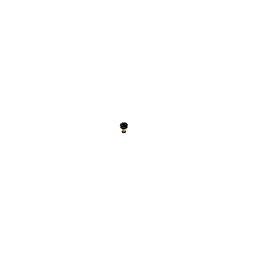
shadowmask_LN_evap_fixture (Autodesk Fusion 360 archive; units mm, degrees)
design "pelco_SEMclip_simplified_bolt"
Autodesk Fusion 360 part; units mm, degrees
sketch "Sketch3" plane through (0, 0, 1.43) normal (0, 0, 1) x (-1, 0, 0)
  circle A0 centre (0, 0) radius 1.895
  line L0 (-2, -0.3) -> (2, -0.3)
  line L1 (2, -0.3) -> (2, 0.3)
  line L2 (2, 0.3) -> (-2, 0.3)
  line L3 (-2, 0.3) -> (-2, -0.3)
  line L4 (-2, -0.3) -> (2, 0.3) construction
  line L5 (2, -0.3) -> (-2, 0.3) construction
  constraint horizontal L0
  constraint perpendicular L0 L1
  constraint parallel L0 L2
  constraint parallel L1 L3
  constraint coincident L4 A0.centre
  constraint coincident L5 A0.centre
  constraint coincident A0.centre origin
sketch "Sketch1" plane through (0, 0, 0.2) normal (0, 0, 1) x (-1, 0, 0)
  line L0 (1.6, -1.9) -> (1.6, -0.0323)
  line L1 (1.6, -0.0323) -> (1.5997, -0.0323)
  arc A0 (1.5997, -0.0323) -> (-1.5997, -0.0323) centre (0, 0) ccw
  line L2 (-1.5997, -0.0323) -> (-1.6, -0.0323)
  line L3 (-1.6, -0.0323) -> (-1.6, -1.9)
  line L4 (-1.6, -1.9) -> (1.6, -1.9)
  circle A1 centre (0, 0) radius 1.05
  circle A2 centre (0, 0) radius 1.895
  dimension "d39" = 3.79
  constraint concentric A0 A2
  measures "d39" diameter of A2
extrude "Extrude1" add sketch "Sketch1" along normal blind 1.23 contours L0 A0 L3 A2 | L0 A0 L3 A2 | A1
sketch "Sketch2" plane through (0, 0, 0.2) normal (0, 0, -1) x (1, 0, 0)
  circle A0 centre (0, 0) radius 1.895
  circle A1 centre (0, 0) radius 1
  dimension "d42" = 2
  constraint coincident A0.centre A1.centre
  measures "d42" diameter of A1
extrude "Extrude2" add sketch "Sketch2" along normal blind 3.5 contours A1
extrude "Extrude3" cut sketch "Sketch3" against normal blind 1 contours A0 L0 L2

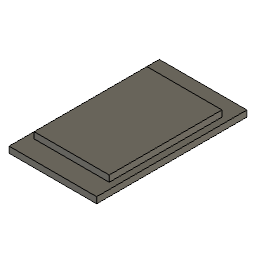
design "6x9_12x7_300um_sm_flipchip_assemb"
Autodesk Fusion 360 part; units mm, degrees
sketch "Sketch1" plane through (0, 0, 0) normal (0, 0, 1) x (1, 0, 0)
  line L0 (3.5, 6) -> (-3.5, 6)
  line L1 (-3.5, 6) -> (-3.5, -6)
  line L2 (-3.5, -6) -> (3.5, -6)
  line L3 (3.5, -6) -> (3.5, 6)
  line L4 (3.5, 6) -> (-3.5, -6) construction
  line L5 (-3.5, 6) -> (3.5, -6) construction
  dimension "d1" = 7
  dimension "d2" = 12
  constraint horizontal L0
  constraint perpendicular L0 L1
  constraint parallel L0 L2
  constraint parallel L1 L3
  constraint coincident L4 origin
  constraint coincident L5 origin
  measures "d1" distance of L1 L3
  measures "d2" distance of L0 L2
extrude "Extrude1" add sketch "Sketch1" along normal blind 0.5 makes body 1
sketch "Sketch2" plane through (0, 0, 0) normal (0, 0, -1) x (1, 0, 0)
  line L0 (3.5, -6) -> (3.5, 6)
  line L1 (3.5, 6) -> (-3.5, 6)
  line L2 (-3.5, 6) -> (-3.5, -6)
  line L3 (-3.5, -6) -> (3.5, -6)
  line L4 (2, 2.5) -> (-2, 2.5)
  line L5 (-2, 2.5) -> (-2, -2.5)
  line L6 (-2, -2.5) -> (2, -2.5)
  line L7 (2, -2.5) -> (2, 2.5)
  line L8 (2, 2.5) -> (-2, -2.5) construction
  line L9 (-2, 2.5) -> (2, -2.5) construction
  dimension "d6" = 4
  dimension "d7" = 5
  constraint horizontal L4
  constraint perpendicular L4 L5
  constraint parallel L4 L6
  constraint parallel L5 L7
  constraint coincident L8 origin
  constraint coincident L9 origin
  measures "d6" distance of L5 L7
  measures "d7" distance of L4 L6
extrude "Extrude2" cut sketch "Sketch2" against normal blind 0.25 contours L4 L5 L6 L7 bodies 1
chamfer "Chamfer2" distance 0.25 angle 45 4 edges at (-2, 0, 0.25) (0, 2.5, 0.25) (0, -2.5, 0.25) (2, 0, 0.25) on bodies 1
sketch "Sketch3" plane through (0, 0, 0.5) normal (0, 0, 1) x (-1, 0, 0)
  line L0 (-3.5, -6) -> (3.5, -6)
  line L1 (3.5, -6) -> (3.5, 6)
  line L2 (3.5, 6) -> (-3.5, 6)
  line L3 (-3.5, 6) -> (-3.5, -6)
  line L4 (-3, -4.5) -> (3, -4.5)
  line L5 (3, -4.5) -> (3, 4.5)
  line L6 (3, 4.5) -> (-3, 4.5)
  line L7 (-3, 4.5) -> (-3, -4.5)
  line L8 (-3, -4.5) -> (3, 4.5) construction
  line L9 (3, -4.5) -> (-3, 4.5) construction
  dimension "d11" = 9
  dimension "d12" = 6
  constraint horizontal L4
  constraint perpendicular L4 L5
  constraint parallel L4 L6
  constraint parallel L5 L7
  constraint coincident L8 origin
  constraint coincident L9 origin
  measures "d11" distance of L4.end L5.end
  measures "d12" distance of L4.start L4.end
extrude "Extrude3" add sketch "Sketch3" along normal blind 0.5 contours L4 L5 L6 L7 bodies 1
sketch "Sketch4" plane through (0, 0, 0.25) normal (0, 0, -1) x (1, 0, 0)
  line L0 (-1.75, -2.25) -> (1.75, -2.25)
  line L1 (1.75, -2.25) -> (1.75, 2.25)
  line L2 (1.75, 2.25) -> (-1.75, 2.25)
  line L3 (-1.75, 2.25) -> (-1.75, -2.25)
  line L4 (1.75, -2.25) -> (-1.75, -2.25)
  line L5 (-1.75, -2.25) -> (-1.75, 2.25)
  line L6 (-1.75, 2.25) -> (1.75, 2.25)
  line L7 (1.75, 2.25) -> (1.75, -2.25)
  constraint horizontal L4
  constraint vertical L5
  constraint horizontal L6
  constraint vertical L7
  constraint coincident L2.end L3.start
  constraint coincident L0.end L1.start
extrude "Extrude4" add sketch "Sketch4" along normal blind 0.01 from surface at 0.01 separate body makes body 2

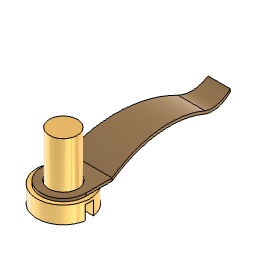
design "pelco_SEMclip_simplified_flipped"
Autodesk Fusion 360 part; units mm, degrees
sketch "Sketch1" plane through (0, 0, 0) normal (0, 0, 1) x (1, 0, 0)
  circle A0 centre (0, 0) radius 1.05
  circle A1 centre (0, 0) radius 1.6
  line L0 (-1.6, 1.9) -> (1.6, 1.9)
  line L1 (1.6, 1.9) -> (1.6, 0.0323)
  line L2 (1.6, 0.0323) -> (-1.6, 0.0323)
  line L3 (-1.6, 0.0323) -> (-1.6, 1.9)
  line L4 (-0.8, 11.2) -> (0.8, 11.2)
  line L5 (0.8, 11.2) -> (0.8, 10.2)
  line L6 (0.8, 10.2) -> (-0.8, 10.2)
  line L7 (-0.8, 10.2) -> (-0.8, 11.2)
  line L8 (-1.6, 1.9) -> (-0.8, 11.2)
  line L9 (0.8, 11.2) -> (1.6, 1.9)
  dimension "d1" = 2.1
  dimension "d2" = 3.2
  dimension "d3" = 1.6
  dimension "d4" = 1.6
  dimension "d5" = 1.9
  dimension "d6" = 0.8
  dimension "d7" = 0.8
  dimension "d8" = 11.2
  constraint coincident A0.centre A1.centre
  constraint concentric A0 A1
  constraint horizontal L0
  constraint vertical L1
  constraint horizontal L2
  constraint vertical L3
  constraint horizontal L4
  constraint vertical L5
  constraint horizontal L6
  constraint vertical L7
  measures "d1" diameter of A0
  measures "d2" diameter of A1
  measures "d3" distance of A0.centre L3
  measures "d4" distance of A0.centre L1
  measures "d5" distance of A0.centre L0
  measures "d6" distance of A0.centre L7
  measures "d7" distance of A0.centre L5
  measures "d8" distance of A0.centre L4
extrude "Extrude1" add sketch "Sketch1" along normal blind 1.3 contours A0 A1 L2 | A0 A1 L2 | A1 L0 L1 L3 | L0 L5 L6 L7 L8 L9 | L4 L5 L6 L7 makes body 1
sketch "Sketch3" plane through (0, 0, 0) normal (1, 0, 0) x (0, 1, 0)
sketch "Sketch4" plane through (0, 0, 0) normal (1, 0, 0) x (0, 1, 0)
  line L0 (-1.6, 1.3) -> (1.9, 1.3)
  line L1 (1.9, 1.3) -> (1.9, 0.2)
  line L2 (1.9, 0.2) -> (-1.6, 0.2)
  line L3 (-1.6, 0.2) -> (-1.6, 1.3)
  line L4 (1.9, 1.3) -> (0.0323, 1.3)
  arc A0 (9.2226, 0.2) -> (11.2, 0.5) centre (9.961, 2) ccw
  line L5 (0.0323, 0) -> (1.9, 0)
  line L6 (11.2, 0) -> (11.2, 1.3)
  arc A1 (9.2226, 0.2) -> (1.9, 0) centre (5.7552, -7) ccw
  arc A2 (9.2226, 0.4) -> (11.2, 0.7) centre (9.961, 2.2) ccw
  arc A3 (9.2226, 0.4) -> (1.9, 0.2) centre (5.7552, -6.8) ccw
  line L7 (11.2, 0.7) -> (11.2, 0.5)
  line L8 (11.2, 0.5) -> (11.2, 0)
  line L9 (11.2, 0) -> (1.9, 0)
  line L10 (1.9, 0) -> (-1.6, 0)
  line L11 (-1.6, 0) -> (-1.6, 0.2)
  line L12 (1.9, 1.3) -> (11.2, 1.3)
  line L13 (11.2, 1.3) -> (11.2, 0.7)
  dimension "d21" = 0.2
  dimension "d24" = 0.5
  dimension "d25" = 0.2
  dimension "d26" = 2
  dimension "d27" = 2
  dimension "d28" = 1.9
  dimension "d29" = 1.6
  dimension "d30" = 1.3
  dimension "d32" = 7
  dimension "d35" = 0.2
  dimension "d36" = 0
  constraint horizontal L0
  constraint vertical L1
  constraint horizontal L2
  constraint vertical L3
  constraint coincident A0.end L6
  constraint coincident L5.end A1.end
  constraint coincident L1 L5.end
  constraint coincident L6.start L8.end
  constraint parallel L9 L10
  constraint coincident L0.end L1.start
  constraint coincident L6.end L12.end
  measures "d21" distance of origin L2
  measures "d24" distance of A0.end L5
  measures "d25" distance of A0.start L5
  measures "d26" distance of A0.start A0.end
  measures "d27" vertical distance of origin A0.centre
  measures "d28" distance of origin L1
  measures "d29" distance of origin L3
  measures "d30" distance of origin L0
  measures "d32" distance of L5 A1.centre
extrude "Extrude3" cut sketch "Sketch4" along normal mid plane 10 contours L0 L1 L2 L3 L4 | L1 L6 A2 A3 L12 L13 | A0 L6 A1 L8 L9 bodies 1
sketch "Sketch1 (2)" plane through (0, 0, 0.2) normal (0, 0, 1) x (-1, 0, 0) in component "bolt"
  line L0 (1.6, -1.9) -> (1.6, -0.0323)
  line L1 (1.6, -0.0323) -> (1.5997, -0.0323)
  arc A0 (1.5997, -0.0323) -> (-1.5997, -0.0323) centre (0, 0) ccw
  line L2 (-1.5997, -0.0323) -> (-1.6, -0.0323)
  line L3 (-1.6, -0.0323) -> (-1.6, -1.9)
  line L4 (-1.6, -1.9) -> (1.6, -1.9)
  circle A1 centre (0, 0) radius 1.05
  circle A2 centre (0, 0) radius 1.895
  dimension "d39" = 3.79
  constraint concentric A0 A2
  measures "d39" diameter of A2
extrude "Extrude1'" add sketch "Sketch1 (2)" along normal blind 1.23 separate body contours L0 A0 L3 A2 | L0 A0 L3 A2 | A1 makes body 2 in component "bolt"
sketch "Sketch2" plane through (0, 0, 0.2) normal (0, 0, -1) x (1, 0, 0) in component "bolt"
  circle A0 centre (0, 0) radius 1.895
  circle A1 centre (0, 0) radius 1
  dimension "d42" = 2
  constraint coincident A0.centre A1.centre
  measures "d42" diameter of A1
extrude "Extrude2" add sketch "Sketch2" along normal blind 3.5 contours A1 bodies 2 in component "bolt"
sketch "Sketch5" plane through (0, 0, 1.43) normal (0, 0, 1) x (-1, 0, 0)
  circle A0 centre (0, 0) radius 1.895
  line L0 (-2, -0.3) -> (2, -0.3)
  line L1 (2, -0.3) -> (2, 0.3)
  line L2 (2, 0.3) -> (-2, 0.3)
  line L3 (-2, 0.3) -> (-2, -0.3)
  line L4 (-2, -0.3) -> (2, 0.3) construction
  line L5 (2, -0.3) -> (-2, 0.3) construction
  constraint horizontal L0
  constraint perpendicular L0 L1
  constraint parallel L0 L2
  constraint parallel L1 L3
  constraint coincident L4 A0.centre
  constraint coincident L5 A0.centre
  constraint coincident A0.centre origin
extrude "Extrude3'" cut sketch "Sketch5" against normal blind 1 contours A0 L0 L2 bodies 2 in component "bolt"
component "bolt" placed x (1, 0, 0) y (0, -1, 0) z (0, 0, -1) at (0, 0, 0.2)
